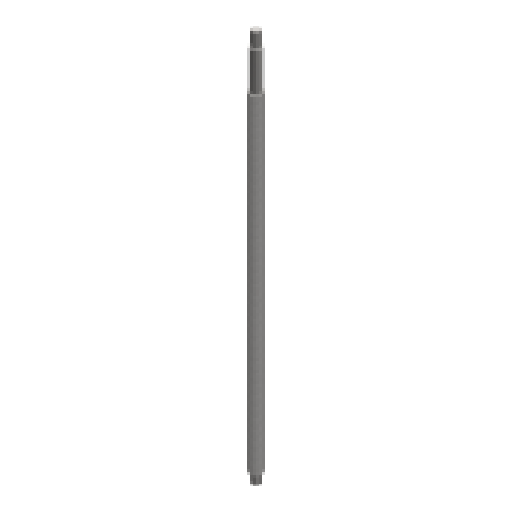
# Autodesk Inventor part: Z Axis Ball Screw
Saved by Autodesk Inventor 2023.2 (Build 272271000, 271)
## iProperties
Created: 2023-02-17
Part Number: Z Axis Ball Screw
Material: Stainless Steel
Document SubType Name: Modeling
Designer: remop
Density: 8 g/cm^3
Appearance: Semi-Polished
Author: remop
Autodesk Inventor part; units mm, degrees
ref_plane "YZ Plane" through (0, 0, 0) normal (1, 0, 0) x (0, 1, 0)
ref_plane "XZ Plane" through (0, 0, 0) normal (0, 1, 0) x (-1, 0, 0)
ref_plane "XY Plane" through (0, 0, 0) normal (0, 0, 1) x (1, 0, 0)
sketch "Sketch1" plane through (0, 0, 0) normal (0, 0, 1) x (1, 0, 0)
  line L0 (0, 0) -> (0, 400)
  line L1 (0, 400) -> (4, 400)
  line L2 (4, 400) -> (4, 385)
  line L3 (4, 385) -> (5, 385)
  line L4 (5, 385) -> (5, 346)
  line L5 (5, 346) -> (6, 346)
  line L6 (6, 346) -> (6, 10)
  line L7 (6, 10) -> (4, 10)
  line L8 (4, 10) -> (4, 0)
  line L9 (4, 0) -> (0, 0)
  dimension "d0" = 400
  dimension "d1" = 8
  dimension "d2" = 10
  dimension "d3" = 12
  dimension "d4" = 10
  dimension "d5" = 8
  dimension "d6" = 15
  dimension "d7" = 39
  constraints: 20 end point, 8 perpendicular, 1 horizontal, 1 vertical
  measures "d0" distance of L0.start L0.end
  measures "d1" diameter of L8 L0
  measures "d2" distance of L7.end L8.end
  measures "d3" diameter of L6 L0
  measures "d4" diameter of L4 L0
  measures "d5" diameter of L2 L0
  measures "d6" distance of L1.end L2.end
  measures "d7" distance of L3.end L4.end
revolve "Revolution1" add sketch "Sketch1" angle 360 about axis through (0, 0, 0) along (0, 1, 0)
thread "Thread1" size "TR12x2" class "7e" standard "ISO Metric Trapezoidal Threads" full length
body "Solid1"
